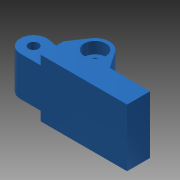
# Autodesk Inventor part: Infill3DIdler
Saved by Autodesk Inventor 2015 SP1 (Build 190203100, 203)
## iProperties
Created: 2015-04-27
Part Number: Infill3DIdler
Material: Generic
Document SubType Name: Modeling
Designer: Jack
Density: 1 g/cm^3
Appearance: Cyan
Author: Jack
Autodesk Inventor part; units mm, degrees
ref_plane "YZ Plane" through (0, 0, 0) normal (1, 0, 0) x (0, 1, 0)
ref_plane "XZ Plane" through (0, 0, 0) normal (0, 1, 0) x (-1, 0, 0)
ref_plane "XY Plane" through (0, 0, 0) normal (0, 0, 1) x (1, 0, 0)
sketch "Sketch1" plane through (0, 0, 0) normal (0, 0, 1) x (1, 0, 0)
  line L0 (0, 0) -> (30, 0)
  line L1 (30, 0) -> (30, 8)
  arc A0 (12.1409, 13.7024) -> (3.8591, 13.7024) centre (8, 10.9) ccw
  line L2 (30, 8) -> (16, 8)
  line L3 (0, 0) -> (0, 8)
  line L4 (0, 8) -> (3.8591, 13.7024)
  line L5 (12.1409, 13.7024) -> (16, 8)
  dimension "d0" = 8
  dimension "d1" = 30
  dimension "d2" = 22
  dimension "d3" = 10.9
  dimension "d4" = 10
  dimension "d5" = 8
  constraints: 12 end point, 2 horizontal, 2 point on circle, 2 tangent, 1 centre point, 1 equal length, 1 perpendicular, 1 vertical
  measures "d0" distance of L0.end L1.end
  measures "d1" distance of L0.start L0.end
  measures "d2" horizontal distance of L1.end A0.centre
  measures "d3" distance from line of L0 A0.centre
  measures "d4" diameter of A0
  measures "d5" distance of L0.start L3.end
extrude "Extrusion1" add sketch "Sketch1" along normal blind 20
ref_plane "Work Plane1" through (0, 0, 10) normal (0, 0, 1) x (1, 0, 0)
sketch "Sketch2" plane through (0, 0, 10) normal (0, 0, 1) x (1, 0, 0)
  arc A0 (12.1409, 13.7024) -> (3.8591, 13.7024) centre (8, 10.9) ccw projected
  arc A1 (-6.1752, 9.1255) -> (-7, 0) centre (-7, 4.6) ccw
  line L0 (-6.1752, 9.1255) -> (0, 8)
  line L1 (-7, 0) -> (0, 0)
  line L2 (0, 8) -> (0, 0)
  dimension "d9" = 6.3
  dimension "d10" = 15
  dimension "d11" = 9.2
  constraints: 6 end point, 2 point on circle, 2 tangent, 1 centre point, 1 vertical
  measures "d9" vertical distance of A0.centre A1.centre
  measures "d10" horizontal distance of A1.centre A0.centre
  measures "d11" diameter of A1
extrude "Extrusion2" add sketch "Sketch2" along normal mid plane 13.6
sketch "Sketch3" plane through (0, 0, 16.8) normal (0, 0, 1) x (1, 0, 0)
  arc A0 (-6.1752, 9.1255) -> (-7, 0) centre (-7, 4.6) ccw projected
hole "Hole1" at (-7, 4.6, 16.8) direction (0, 0, -1) diameter 3.5 end through all
sketch "Sketch4" plane through (0, 0, 20) normal (0, 0, 1) x (1, 0, 0)
  arc A0 (12.1409, 13.7024) -> (3.8591, 13.7024) centre (8, 10.9) ccw projected
hole "Hole2" at (8, 10.9, 20) direction (0, 0, -1) diameter 4.5 end through all
ref_plane "Work Plane2" through (0, 0, 10) normal (0, 0, 1) x (1, 0, 0)
sketch "Sketch5" plane through (0, 0, 10) normal (0, 0, 1) x (1, 0, 0)
  circle A0 centre (8, 10.9) radius 2.25 projected
  circle A1 centre (8, 10.9) radius 8
  point P0 (0, 0)
  dimension "d29" = 16
  constraints: 1 centre point, 1 coincident
  measures "d29" diameter of A1
extrude "Extrusion3" cut sketch "Sketch5" along normal mid plane 7
sketch "Sketch6" plane through (0, 0, 20) normal (0, 0, 1) x (1, 0, 0)
  circle A0 centre (8, 10.9) radius 2.25 projected
hole "Hole3" at (8, 10.9, 20) direction (0, 0, -1) diameter 7.5 depth 4
sketch "Sketch7" plane through (0, 0, 0) normal (0, 0, -1) x (-1, 0, 0)
  circle A0 centre (-8, 10.9) radius 2.25 projected
  arc A1 (-3.8591, 13.7024) -> (-12.1409, 13.7024) centre (-8, 10.9) ccw projected
  line L0 (-8, 6.6276) -> (-11.7, 8.7638)
  line L1 (-11.7, 8.7638) -> (-11.7, 13.0362)
  line L2 (-11.7, 13.0362) -> (-8, 15.1724)
  line L3 (-8, 15.1724) -> (-4.3, 13.0362)
  line L4 (-4.3, 13.0362) -> (-4.3, 8.7638)
  line L5 (-4.3, 8.7638) -> (-8, 6.6276)
  dimension "d39" = 7.4
  constraints: 12 end point, 1 coincident, 1 vertical, 13 other
  measures "d39" distance between parallel lines of L4 L1
extrude "Extrusion4" cut sketch "Sketch7" against normal blind 3.5
sketch "Sketch8" plane through (0, 0, 6.5) normal (0, 0, 1) x (1, 0, 0)
  circle A0 centre (8, 10.9) radius 2.25 projected
  circle A1 centre (8, 10.9) radius 5
  point P0 (0, 0)
  dimension "d42" = 10
  constraints: 1 centre point, 1 coincident
  measures "d42" diameter of A1
extrude "Extrusion5" add sketch "Sketch8" along normal blind 1
sketch "Sketch9" plane through (0, 0, 13.5) normal (0, 0, -1) x (-1, 0, 0)
  arc A0 (-3.8591, 13.7024) -> (-12.1409, 13.7024) centre (-8, 10.9) ccw projected
  circle A1 centre (-8, 10.9) radius 2.25 projected
  circle A2 centre (-8, 10.9) radius 5
  point P0 (0, 0)
  constraints: 1 centre point, 1 coincident, 1 concentric
extrude "Extrusion6" add sketch "Sketch9" along normal blind 1
chamfer "Chamfer1" distance 1 angle 45 2 edges at (3, 10.9, 7.5) (13, 10.9, 12.5)
body "Solid1"
